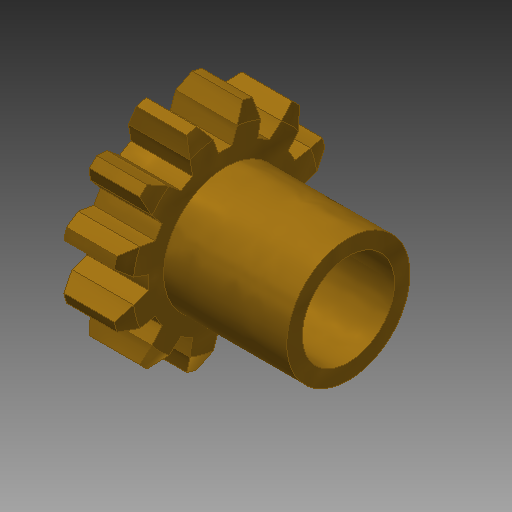
# Autodesk Inventor part: Zahnrad Messing z12
Saved by Autodesk Inventor 2019.1 (Build 231200000, 200)
## iProperties
Category: PARTsolutions
Company: MAEDLER
Created: 2018-08-20
Part Number: Zahnrad Messing z12
Material: Messing, weicher Gelbton, geschweißt
Catalog Web Link: www.cadenas.de
Description: Stzr Messing Ms58-Spur Gears, Brass, Helical Tooth Right Hand, with one-sided hub
Vendor: MAEDLER
Document SubType Name: Modeling
Designer: psadmin
Manufacturer: MAEDLER
Mass: 0.7 g
Surface Area: 2.04431 cm^2
Volume: 0.0867405 cm^3
Density: 8.07005 g/cm^3
Appearance: Schweißnaht - Messing
PSOL_IDENT_0: {$CADENAS_DATA\23d-libs\maedler\antriebselemente\stirnzahnraeder\stirnzahnraeder_messing\stzr_messin
PSOL_IDENT_1: g_ms58.prj},204 {VTYP=3D},{NB=Stzr Messing Ms58 26101200},{LINA=Stzr Messing Ms58 26101200},{NN=Stzr
PSOL_IDENT_2: Messing Ms58},{DATE=03.08.2018 09:08:56},{GEOMDATE=26.07.2018 09:15:44},{VERSION=},{LINEID=190},{WB
PSOL_IDENT_3: VAR=},{WBNUMERIC=}  {NB=Stzr Messing Ms58 26101200},{LINA=Stzr Messing Ms58 26101200},{KT=DUMMY},{AR
PSOL_IDENT_4: TNR=26101200},{WST=Messing (Ms58)},{M=0.5},{Z=12},{PDF=PDF Katalogseite},{B1=2.0},{DA=7.00},{D=6.00}
PSOL_IDENT_5: ,{NL=4},{ND=4},{B=2.00},{MD=0.6},{GEW=0.700}
NN: Stzr Messing Ms58
NT: Spur Gears, Brass, Helical Tooth Right Hand, with one-sided hub
NB: Stzr Messing Ms58 26101200
NBSYN: Stzr Messing Ms58 $ARTNR.
LINA: Stzr Messing Ms58 26101200
ARTNR: 26101200
WST: Messing (Ms58)
M: 0.5
Z: 12
PDF: PDF Katalogseite
B1: 2
DA: 7
D: 6
NL: 4
ND: 4
B: 2
MD: 0.6
GEW: 0.7
SUPPLIER: MAEDLER
ARTICLENO: Stzr Messing Ms58 26101200
BOMINFO: Stzr Messing Ms58 26101200
CREATOR: CADENAS GmbH
Title: Stzr Messing Ms58 26101200
Author: Cadenas PARTsolutions
Comments: Spur Gears, Brass, Helical Tooth Right Hand, with one-sided hub
Autodesk Inventor part; units mm, degrees
ref_plane "YZ Plane" through (0, 0, 0) normal (1, 0, 0) x (0, 1, 0)
ref_plane "XZ Plane" through (0, 0, 0) normal (0, 1, 0) x (-1, 0, 0)
ref_plane "XY Plane" through (0, 0, 0) normal (0, 0, 1) x (1, 0, 0)
sketch "Skizze_1" plane through (0, 0, 0) normal (0, 0, 1) x (1, 0, 0)
  line L0 (6, 0) -> (0, 0)
  line L1 (0, 1) -> (6, 1)
  line L2 (6, 1) -> (6, 2)
  line L3 (6, 2) -> (2, 2)
  line L4 (2, 2) -> (2, 3)
  line L5 (2, 3) -> (1, 5.7475)
  line L6 (1, 5.7475) -> (0, 3)
  line L7 (0, 3) -> (0, 1)
  constraints: 16 end point
revolve "Revolution1" add sketch "Skizze_1" angle 360 about axis through (6, 0, 0) along (1, 0, 0)
sketch "Skizze_2" plane through (2, 0, 0) normal (1, 0, 0) x (0, 0, -1)
  circle A0 centre (0, 0) radius 10.5
  arc A1 (-3.42, -0.7439) -> (-3.3338, -1.0658) centre (0, 0) ccw
  line L0 (-3.3338, -1.0658) -> (-2.7725, -1.1459)
  line L1 (-2.7725, -1.1459) -> (-2.2658, -1.0565)
  arc A2 (-2.2658, -1.0565) -> (-2.0479, -1.4339) centre (0, 0) ccw
  line L2 (-2.0479, -1.4339) -> (-2.3786, -1.8281)
  line L3 (-2.3786, -1.8281) -> (-2.5899, -2.3542)
  arc A3 (-2.5899, -2.3542) -> (-2.3542, -2.5899) centre (0, 0) ccw
  line L4 (-2.3542, -2.5899) -> (-1.8281, -2.3786)
  line L5 (-1.8281, -2.3786) -> (-1.4339, -2.0479)
  arc A4 (-1.4339, -2.0479) -> (-1.0565, -2.2658) centre (0, 0) ccw
  line L6 (-1.0565, -2.2658) -> (-1.1459, -2.7725)
  line L7 (-1.1459, -2.7725) -> (-1.0658, -3.3338)
  arc A5 (-1.0658, -3.3338) -> (-0.7439, -3.42) centre (0, 0) ccw
  line L8 (-0.7439, -3.42) -> (-0.3939, -2.974)
  line L9 (-0.3939, -2.974) -> (-0.2179, -2.4905)
  arc A6 (-0.2179, -2.4905) -> (0.2179, -2.4905) centre (0, 0) ccw
  line L10 (0.2179, -2.4905) -> (0.3939, -2.974)
  line L11 (0.3939, -2.974) -> (0.7439, -3.42)
  arc A7 (0.7439, -3.42) -> (1.0658, -3.3338) centre (0, 0) ccw
  line L12 (1.0658, -3.3338) -> (1.1459, -2.7725)
  line L13 (1.1459, -2.7725) -> (1.0565, -2.2658)
  arc A8 (1.0565, -2.2658) -> (1.4339, -2.0479) centre (0, 0) ccw
  line L14 (1.4339, -2.0479) -> (1.8281, -2.3786)
  line L15 (1.8281, -2.3786) -> (2.3542, -2.5899)
  arc A9 (2.3542, -2.5899) -> (2.5899, -2.3542) centre (0, 0) ccw
  line L16 (2.5899, -2.3542) -> (2.3786, -1.8281)
  line L17 (2.3786, -1.8281) -> (2.0479, -1.4339)
  arc A10 (2.0479, -1.4339) -> (2.2658, -1.0565) centre (0, 0) ccw
  line L18 (2.2658, -1.0565) -> (2.7725, -1.1459)
  line L19 (2.7725, -1.1459) -> (3.3338, -1.0658)
  arc A11 (3.3338, -1.0658) -> (3.42, -0.7439) centre (0, 0) ccw
  line L20 (3.42, -0.7439) -> (2.974, -0.3939)
  line L21 (2.974, -0.3939) -> (2.4905, -0.2179)
  arc A12 (2.4905, -0.2179) -> (2.4905, 0.2179) centre (0, 0) ccw
  line L22 (2.4905, 0.2179) -> (2.974, 0.3939)
  line L23 (2.974, 0.3939) -> (3.42, 0.7439)
  arc A13 (3.42, 0.7439) -> (3.3338, 1.0658) centre (0, 0) ccw
  line L24 (3.3338, 1.0658) -> (2.7725, 1.1459)
  line L25 (2.7725, 1.1459) -> (2.2658, 1.0565)
  arc A14 (2.2658, 1.0565) -> (2.0479, 1.4339) centre (0, 0) ccw
  line L26 (2.0479, 1.4339) -> (2.3786, 1.8281)
  line L27 (2.3786, 1.8281) -> (2.5899, 2.3542)
  arc A15 (2.5899, 2.3542) -> (2.3542, 2.5899) centre (0, 0) ccw
  line L28 (2.3542, 2.5899) -> (1.8281, 2.3786)
  line L29 (1.8281, 2.3786) -> (1.4339, 2.0479)
  arc A16 (1.4339, 2.0479) -> (1.0565, 2.2658) centre (0, 0) ccw
  line L30 (1.0565, 2.2658) -> (1.1459, 2.7725)
  line L31 (1.1459, 2.7725) -> (1.0658, 3.3338)
  arc A17 (1.0658, 3.3338) -> (0.7439, 3.42) centre (0, 0) ccw
  line L32 (0.7439, 3.42) -> (0.3939, 2.974)
  line L33 (0.3939, 2.974) -> (0.2179, 2.4905)
  arc A18 (0.2179, 2.4905) -> (-0.2179, 2.4905) centre (0, 0) ccw
  line L34 (-0.2179, 2.4905) -> (-0.3939, 2.974)
  line L35 (-0.3939, 2.974) -> (-0.7439, 3.42)
  arc A19 (-0.7439, 3.42) -> (-1.0658, 3.3338) centre (0, 0) ccw
  line L36 (-1.0658, 3.3338) -> (-1.1459, 2.7725)
  line L37 (-1.1459, 2.7725) -> (-1.0565, 2.2658)
  arc A20 (-1.0565, 2.2658) -> (-1.4339, 2.0479) centre (0, 0) ccw
  line L38 (-1.4339, 2.0479) -> (-1.8281, 2.3786)
  line L39 (-1.8281, 2.3786) -> (-2.3542, 2.5899)
  arc A21 (-2.3542, 2.5899) -> (-2.5899, 2.3542) centre (0, 0) ccw
  line L40 (-2.5899, 2.3542) -> (-2.3786, 1.8281)
  line L41 (-2.3786, 1.8281) -> (-2.0479, 1.4339)
  arc A22 (-2.0479, 1.4339) -> (-2.2658, 1.0565) centre (0, 0) ccw
  line L42 (-2.2658, 1.0565) -> (-2.7725, 1.1459)
  line L43 (-2.7725, 1.1459) -> (-3.3338, 1.0658)
  arc A23 (-3.3338, 1.0658) -> (-3.42, 0.7439) centre (0, 0) ccw
  line L44 (-3.42, 0.7439) -> (-2.974, 0.3939)
  line L45 (-2.974, 0.3939) -> (-2.4905, 0.2179)
  arc A24 (-2.4905, 0.2179) -> (-2.4905, -0.2179) centre (0, 0) ccw
  line L46 (-2.4905, -0.2179) -> (-2.974, -0.3939)
  line L47 (-2.974, -0.3939) -> (-3.42, -0.7439)
  constraints: 96 end point, 48 point on circle, 25 centre point
extrude "Extrusion1" cut sketch "Skizze_2" along normal mid plane 12
sketch "Skizze3" plane through (0, 0, 0) normal (-1, 0, 0) x (0, 0, 1)
  circle A0 centre (0, 0) radius 2 projected
  constraints: 1 coincident
hole "Bohrung1" at (0, 0, 0) direction (1, 0, 0) diameter 3 end through all
body "Solid1"
